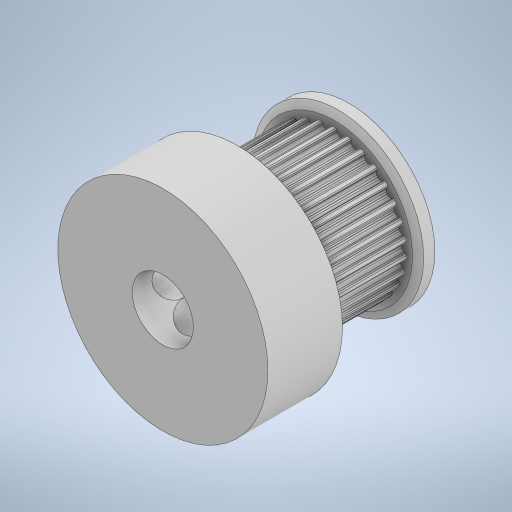
# Autodesk Inventor part: motor-pulley-high-torque
Saved by Autodesk Inventor 2024 (Build 280153000, 153)
## iProperties
Created: 2020-03-26
Part Number: motor-pulley-high-torque
Material: Generic
Document SubType Name: Modeling
Designer: Tyrone.Burcombe
Density: 1 g/cm^3
Appearance: Default
NumTeeth: 31,416 ul
ToothPitch: 2.000 mm
PulleyDia: 20,000 mm
ToothAngle: 11,46 deg
TransOffsetAngle: 2,29 deg
ShoulderRadius: 0.150 mm
RootRadius: 0.555 mm
TransRadius: 1.000 mm
ToothHeight: 0.750 mm
PLD: 0.254 mm
BeltWidth: 11,000 mm
Author: Tyrone.Burcombe
## iProperties of the stored document pulley-140mm_3DPrint.ipt
Created: 2024-02-22
Part Number: pulley-140mm_3DPrint
Material: Generic
Document SubType Name: Modeling
Designer: MaartenGeorgesBuelen
Density: 1 g/cm^3
Appearance: Default
Author: MaartenGeorgesBuelen
Autodesk Inventor part; units mm, degrees
ref_plane "YZ Plane" through (0, 0, 0) normal (1, 0, 0) x (0, 1, 0)
ref_plane "XZ Plane" through (0, 0, 0) normal (0, 1, 0) x (-1, 0, 0)
ref_plane "XY Plane" through (0, 0, 0) normal (0, 0, 1) x (1, 0, 0)
sketch "Sketch1" plane through (0, 0, 0) normal (0, 0, 1) x (1, 0, 0)
  circle A0 centre (0, 0) radius 10 construction
  circle A1 centre (0, 0) radius 9.746 construction
  circle A2 centre (0, 0) radius 8.996 construction
  line L0 (0, 0) -> (0, 10) construction
  line L1 (0, 0) -> (0.9983, 9.95) construction
  line L2 (0, 0) -> (1.3954, 9.9022) construction
  arc A3 (0.6914, 9.0141) -> (0.8981, 8.9511) centre (0.9535, 9.5033) ccw
  arc A4 (0.3612, 9.6011) -> (0.3969, 9.3814) centre (1.36, 9.6506) ccw
  circle A5 centre (0, 0) radius 9.596 construction
  arc A6 (0.2147, 9.7436) -> (0, 9.746) centre (0, 0) ccw
  arc A7 (0.3612, 9.6011) -> (0.2147, 9.7436) centre (0.2114, 9.5937) ccw
  arc A8 (0.3969, 9.3814) -> (0.6914, 9.0141) centre (0.9748, 9.543) ccw
  arc A9 (-0.8981, 8.9511) -> (-0.6914, 9.0141) centre (-0.9535, 9.5033) ccw
  arc A10 (-0.3969, 9.3814) -> (-0.3612, 9.6011) centre (-1.36, 9.6506) ccw
  arc A11 (0, 9.746) -> (-0.2147, 9.7436) centre (0, 0) ccw
  arc A12 (-0.2147, 9.7436) -> (-0.3612, 9.6011) centre (-0.2114, 9.5937) ccw
  arc A13 (-0.6914, 9.0141) -> (-0.3969, 9.3814) centre (-0.9748, 9.543) ccw
  arc A14 (-0.8981, 8.9511) -> (0.8981, 8.9511) centre (0, 0) ccw
  circle A15 centre (0, 0) radius 4.1
  point P0 (1.7655, 5.0632)
  point P1 (-1.7655, 5.0632)
  dimension "d0" = 20
  dimension "d1" = 5.73
  dimension "d2" = 2.292
  dimension "d3" = 1.004
  dimension "d4" = 0.75
  dimension "d5" = 0.555
  dimension "d6" = 1
  dimension "d7" = 0.15
  dimension "d9" = 0.6
  dimension "d21" = 8.2
  constraints: 27 point on circle, 14 centre point, 9 symmetric about line, 7 coincident, 6 end point, 4 tangent, 2 point on line, 1 vertical, 12 other
  measures "d0" diameter of A0
  measures "d1" angle of L1 L0
  measures "d2" angle of L2 L1
  measures "d5" radius of A3
  measures "d6" radius of A4
  measures "d9" radius of A8
  measures "d21" diameter of A15
extrude "Extrusion1" add sketch "Sketch1" along normal mid plane 11
pattern_circular "Circular Pattern1" count 31 over 360 about axis through (0, 0, 0) along (0, 0, 1) of "Extrusion1"
sketch "Sketch2" plane through (0, 0, 5.5) normal (0, 0, 1) x (1, 0, 0)
  circle A0 centre (0, 0) radius 11.5
  circle A1 centre (0, 0) radius 4.1 projected
  dimension "d15" = 23
  constraints: 1 centre point, 1 coincident
  measures "d15" diameter of A0
extrude "Extrusion2" add sketch "Sketch2" along normal blind 2
chamfer "Chamfer1" distance 1 distance2 0.5 1 edges at (-11.5, 0, 5.5) measured on face at (-11, 0, 5.5)
mirror "Mirror1" about plane through (0, 0, 0) normal (0, 0, 1) of "Extrusion2", "Chamfer1"
sketch "Sketch12" plane through (0, 0, 7.5) normal (0, 0, 1) x (1, 0, 0)
  circle A0 centre (0, 0) radius 11.5 projected
  circle A1 centre (0, 0) radius 4.1 projected
  circle A2 centre (0, 0) radius 14.1
  dimension "d42" = 10
  constraints: 1 centre point
  measures "d42" radial gap between concentric circles of A1 A2
extrude "Extrusion8" add sketch "Sketch12" along normal blind 9 contours A0 | A2
sketch "Sketch14" plane through (0, 0, 16.5) normal (0, 0, 1) x (1, 0, 0)
  circle A0 centre (0, 0) radius 10.1 projected
  line L0 (0, -10.1) -> (0, 10.1)
  line L1 (10.1, 0) -> (-10.1, 0)
  constraints: 4 end point, 4 point on circle, 1 perpendicular, 1 vertical
ref_plane "Work Plane8" through (0, -10.1, 16.5) normal (1, 0, 0) x (0, 1, 0)
ref_plane "Work Plane9" through (10.1, 0, 16.5) normal (0, 1, 0) x (-1, 0, 0)
ref_plane "Work Plane10" through (-14.1, 0, 7.5) normal (1, 0, 0) x (0, 1, 0)
ref_plane "Work Plane11" through (0, -14.1, 7.5) normal (0, 1, 0) x (-1, 0, 0)
sketch "Sketch15" plane through (-14.1, 0, 7.5) normal (1, 0, 0) x (0, 1, 0)
  line L0 (14.1, 9) -> (-14.1, 9) projected
  circle A0 centre (0, 4.5) radius 2.875
  line L1 (-14.1, 13.8) -> (-14.1, -19.8) projected
  point P0 (0, -7.5)
  point P1 (-10.1, 0)
  point P2 (10.1, 0)
  point P3 (-14.1, -19.8)
  dimension "d51" = 5.75
  dimension "d52" = 4.5
  dimension "d61" = 14.1
  constraints: 1 centre point, 1 other
  measures "d51" diameter of A0
  measures "d52" distance from line of A0.centre L0
extrude "Extrusion10" cut sketch "Sketch15" along normal up to surface round surface about axis through (0, 0, 0) along (0, 0, 1) radius 4.1 far side no
sketch "Sketch16" plane through (0, -14.1, 7.5) normal (0, 1, 0) x (-1, 0, 0)
  line L0 (14.1, 0) -> (14.1, 9) projected
  line L1 (-14.1, 0) -> (-14.1, 9) projected
  line L2 (14.1, 9) -> (-14.1, 9)
  line L3 (-14.1, 9) -> (-14.1, 0)
  line L4 (-14.1, 0) -> (14.1, 0)
  line L5 (14.1, 0) -> (14.1, 9)
  circle A0 centre (0, 4.5) radius 2.9
  point P0 (0, -7.5)
  dimension "d57" = 5.8
  constraints: 8 end point, 2 parallel, 2 point on line, 1 centre point, 1 horizontal, 1 perpendicular
  measures "d57" diameter of A0
extrude "Extrusion11" cut sketch "Sketch16" along normal up to surface contours A0 round surface about axis through (0, 0, 0) along (0, 0, 1) radius 4.1 far side no
move faces "Move1" translate (0, 0, 1) faces at (10.6301, -1.1248, 16.5)
equation "\"d0\" = PulleyDia"
equation "\"d1\" = 0.5 * ToothAngle"
equation "\"d2\" = TransOffsetAngle"
equation "\"d3\" = PLD + ToothHeight"
equation "\"d4\" = ToothHeight"
equation "\"d5\" = RootRadius"
equation "\"d6\" = TransRadius"
equation "\"d7\" = ShoulderRadius"
equation "\"d10\" = BeltWidth"
equation "\"d12\" = NumTeeth"
equation "\"NumTeeth\" = 31.4159"
equation "\"ToothPitch\" = 2"
equation "\"PulleyDia\" = 20"
equation "\"TransOffsetAngle\" = 0.2 * ToothAngle"
equation "\"ShoulderRadius\" = 0.15"
equation "\"RootRadius\" = 0.555"
equation "\"TransRadius\" = 1"
equation "\"ToothHeight\" = 0.75"
equation "\"PLD\" = 0.254"
equation "\"BeltWidth\" = 11"
equation "\"ToothAngle\" = 11.459156deg"
body "Solid1"
